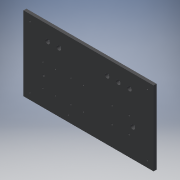
# Autodesk Inventor part: Base2
Saved by Autodesk Inventor 2016 SP1 (Build 200210100, 210)
## iProperties
Created: 2015-09-24
Part Number: Base2
Material: PVC, non plastifié
Document SubType Name: Modeling
Designer: sd
Density: 1.4 g/cm^3
Appearance: Gris
Mass: 783.12 g
Surface Area: 1491.46 cm^2
Volume: 559.372 cm^3
Author: sd
Autodesk Inventor part; units mm, degrees
ref_plane "YZ Plane" through (0, 0, 0) normal (1, 0, 0) x (0, 1, 0)
ref_plane "XZ Plane" through (0, 0, 0) normal (0, 1, 0) x (-1, 0, 0)
ref_plane "XY Plane" through (0, 0, 0) normal (0, 0, 1) x (1, 0, 0)
sketch "Esquisse1" plane through (0, 0, 0) normal (0, 1, 0) x (-1, 0, 0)
  line L0 (-175, 100) -> (175, 100)
  line L1 (175, 100) -> (175, -100)
  line L2 (175, -100) -> (-175, -100)
  line L3 (-175, -100) -> (-175, 100)
  point P0 (0, 0)
  dimension "d0" = 350
  dimension "d1" = 200
  dimension "d93" = 175
  dimension "d94" = 100
  constraints: 8 end point, 2 parallel, 1 horizontal, 1 perpendicular
  measures "d0" distance of L0.start L0.end
  measures "d1" distance of L2.end L0.start
  measures "d93" horizontal distance of point (0, 0) L1.end
  measures "d94" distance from line of point (0, 0) L2
extrude "Extrusion1" add sketch "Esquisse1" along normal blind 8
sketch "Esquisse2" plane through (0, 8, 0) normal (0, 1, 0) x (1, 0, 0)
  line L0 (175, -100) -> (175, 100) projected
  circle A0 centre (109, 46.5) radius 2.25
  circle A1 centre (63, 46.5) radius 2.25
  circle A2 centre (109, 2.5) radius 2.25
  circle A3 centre (63, 2.5) radius 2.25
  line L1 (-175, -100) -> (175, -100) projected
  point P0 (0, 0)
  dimension "d4" = 4.5
  dimension "d5" = 4.5
  dimension "d6" = 4.5
  dimension "d7" = 4.5
  dimension "d14" = 66
  dimension "d15" = 66
  dimension "d46" = 112
  dimension "d47" = 112
  dimension "d48" = 146.5
  dimension "d49" = 146.5
  dimension "d50" = 102.5
  dimension "d51" = 102.5
  constraints: 4 centre point
  measures "d4" diameter of A1
  measures "d5" diameter of A0
  measures "d6" diameter of A2
  measures "d7" diameter of A3
  measures "d14" distance from line of L0 A0.centre
  measures "d15" distance from line of L0 A2.centre
  measures "d46" distance from line of L0 A3.centre
  measures "d47" distance from line of L0 A1.centre
  measures "d48" distance from line of L1 A0.centre
  measures "d49" distance from line of L1 A1.centre
  measures "d50" distance from line of L1 A2.centre
  measures "d51" distance from line of L1 A3.centre
extrude "Extrusion2" cut sketch "Esquisse2" against normal through all
sketch "Esquisse3" plane through (0, 8, 0) normal (0, 1, 0) x (1, 0, 0)
  circle A0 centre (63, 46.5) radius 2.25 projected
  circle A1 centre (63, 2.5) radius 2.25 projected
  line L0 (175, 100) -> (-175, 100) projected
  circle A2 centre (-14, 55.5) radius 2
  circle A3 centre (-48, 55.5) radius 2
  circle A4 centre (-89.1, 55.5) radius 2
  circle A5 centre (-123.1, 55.5) radius 2
  circle A6 centre (-123.1, -6.5) radius 2
  circle A7 centre (-89.1, -6.5) radius 2
  circle A8 centre (-48, -6.5) radius 2
  circle A9 centre (-14, -6.5) radius 2
  point P0 (0, 0)
  dimension "d18" = 4
  dimension "d19" = 4
  dimension "d20" = 4
  dimension "d21" = 4
  dimension "d22" = 4
  dimension "d23" = 4
  dimension "d24" = 4
  dimension "d25" = 4
  dimension "d26" = 62
  dimension "d27" = 62
  dimension "d28" = 62
  dimension "d29" = 62
  dimension "d30" = 34
  dimension "d31" = 34
  dimension "d32" = 34
  dimension "d33" = 34
  dimension "d34" = 41.1
  dimension "d35" = 41.1
  dimension "d36" = 77
  dimension "d37" = 77
  dimension "d38" = 53.5
  dimension "d39" = 44
  dimension "d40" = 44.5
  dimension "d41" = 44.5
  dimension "d42" = 44.5
  dimension "d43" = 44.5
  constraints: 8 centre point
  measures "d18" diameter of A5
  measures "d19" diameter of A4
  measures "d20" diameter of A3
  measures "d21" diameter of A2
  measures "d22" diameter of A9
  measures "d23" diameter of A8
  measures "d24" diameter of A7
  measures "d25" diameter of A6
  measures "d26" distance of A9.centre A2.centre
  measures "d27" distance of A8.centre A3.centre
  measures "d28" distance of A7.centre A4.centre
  measures "d29" distance of A6.centre A5.centre
  measures "d30" distance of A2.centre A3.centre
  measures "d31" distance of A9.centre A8.centre
  measures "d32" distance of A5.centre A4.centre
  measures "d33" distance of A7.centre A6.centre
  measures "d34" distance of A3.centre A4.centre
  measures "d35" distance of A8.centre A7.centre
  measures "d36" horizontal distance of A0.centre A2.centre
  measures "d37" horizontal distance of A1.centre A9.centre
  measures "d38" distance from line of L0 A0.centre
  measures "d39" distance of A1.centre A0.centre
  measures "d40" distance from line of A2.centre L0
  measures "d41" distance from line of L0 A3.centre
  measures "d42" distance from line of L0 A4.centre
  measures "d43" distance from line of L0 A5.centre
extrude "Extrusion3" cut sketch "Esquisse3" against normal through all contours A2 | A3 | A4 | A5 | A6 | A7 | A8 | A9
sketch "Esquisse4" plane through (0, 8, 0) normal (0, 1, 0) x (1, 0, 0)
  circle A0 centre (-121.1, 24.5) radius 3
  circle A1 centre (119, 24.5) radius 6
  circle A2 centre (158, -83) radius 2
  circle A3 centre (158, 83) radius 2
  circle A4 centre (-158, 83) radius 2
  circle A5 centre (-158, -83) radius 2.2714
  circle A6 centre (-110, -60) radius 6
  circle A7 centre (-80, -60) radius 6
  circle A8 centre (50, -60) radius 6
  circle A9 centre (80, -60) radius 6
  circle A10 centre (110, -60) radius 6
  circle A11 centre (-55, 83) radius 2
  line L0 (175, -100) -> (175, 100) projected
  line L1 (-175, 100) -> (-175, -100) projected
  line L2 (175, 100) -> (-175, 100) projected
  line L3 (-175, -100) -> (175, -100) projected
  circle A12 centre (-123.1, 55.5) radius 2 projected
  circle A13 centre (-123.1, -6.5) radius 2 projected
  circle A14 centre (109, 2.5) radius 2.25 projected
  circle A15 centre (109, 46.5) radius 2.25 projected
  point P0 (0, 0)
  dimension "d52" = 4
  dimension "d53" = 4.5428
  dimension "d54" = 4
  dimension "d56" = 4
  dimension "d57" = 6
  dimension "d58" = 12
  dimension "d59" = 17
  dimension "d60" = 17
  dimension "d61" = 17
  dimension "d62" = 17
  dimension "d63" = 17
  dimension "d64" = 17
  dimension "d65" = 17
  dimension "d66" = 4
  dimension "d67" = 17
  dimension "d68" = 2
  dimension "d69" = 31
  dimension "d70" = 62
  dimension "d71" = 17
  dimension "d72" = 120
  dimension "d73" = 44
  dimension "d74" = 22
  dimension "d75" = 10
  dimension "d76" = 30
  dimension "d77" = 12
  dimension "d78" = 12
  dimension "d79" = 12
  dimension "d80" = 12
  dimension "d81" = 12
  dimension "d82" = 30
  dimension "d83" = 30
  dimension "d84" = 40
  dimension "d85" = 40
  dimension "d86" = 40
  dimension "d87" = 65
  dimension "d88" = 40
  dimension "d89" = 40
  dimension "d90" = 130
  constraints: 12 centre point
  measures "d52" diameter of A4
  measures "d53" diameter of A5
  measures "d54" diameter of A3
  measures "d56" diameter of A11
  measures "d57" diameter of A0
  measures "d58" diameter of A1
  measures "d59" distance from line of L1 A4.centre
  measures "d60" distance from line of L2 A4.centre
  measures "d61" distance from line of L2 A3.centre
  measures "d62" distance from line of L0 A3.centre
  measures "d63" distance from line of L1 A5.centre
  measures "d64" distance from line of L3 A5.centre
  measures "d65" distance from line of L3 A2.centre
  measures "d66" diameter of A2
  measures "d67" distance from line of L0 A2.centre
  measures "d68" horizontal distance of A12.centre A0.centre
  measures "d69" vertical distance of A12.centre A0.centre
  measures "d70" distance of A13.centre A12.centre
  measures "d71" distance from line of L2 A11.centre
  measures "d72" distance from line of L1 A11.centre
  measures "d73" distance of A14.centre A15.centre
  measures "d74" vertical distance of A1.centre A15.centre
  measures "d75" horizontal distance of A1.centre A15.centre
  measures "d76" distance of A7.centre A6.centre
  measures "d77" diameter of A6
  measures "d78" diameter of A7
  measures "d79" diameter of A8
  measures "d80" diameter of A9
  measures "d81" diameter of A10
  measures "d82" distance of A9.centre A8.centre
  measures "d83" distance of A10.centre A9.centre
  measures "d84" distance from line of L3 A6.centre
  measures "d85" distance from line of L3 A8.centre
  measures "d86" distance from line of L3 A10.centre
  measures "d87" distance from line of L1 A6.centre
  measures "d88" distance from line of L3 A7.centre
  measures "d89" distance from line of L3 A9.centre
  measures "d90" distance of A7.centre A8.centre
extrude "Extrusion4" cut sketch "Esquisse4" against normal blind 10 contours A0 | A1 | A2 | A3 | A4 | A5 | A6 | A7 | A8 | A9 | A10 | A11
equation "\"d93\" = 0.5 * d0"
equation "\"d94\" = 0.5 * d1"
equation "\"d5\" = d4"
equation "\"d6\" = d4"
equation "\"d7\" = d4"
equation "\"d15\" = d14"
equation "\"d46\" = d47"
equation "\"d49\" = d48"
equation "\"d51\" = d50"
equation "\"d19\" = d18"
equation "\"d20\" = d18"
equation "\"d21\" = d18"
equation "\"d22\" = d18"
equation "\"d23\" = d18"
equation "\"d24\" = d18"
equation "\"d25\" = d18"
equation "\"d27\" = d26"
equation "\"d28\" = d26"
equation "\"d29\" = d26"
equation "\"d31\" = d30"
equation "\"d33\" = d32"
equation "\"d35\" = d34"
equation "\"d37\" = d36"
equation "\"d40\" = d38 + 0.5 * d39 - 0.5 * d26"
equation "\"d41\" = d40"
equation "\"d42\" = d40"
equation "\"d43\" = d40"
equation "\"d54\" = d52"
equation "\"d56\" = d52"
equation "\"d60\" = d59"
equation "\"d61\" = d59"
equation "\"d62\" = d59"
equation "\"d63\" = d59"
equation "\"d64\" = d59"
equation "\"d65\" = d59"
equation "\"d66\" = d52"
equation "\"d67\" = d59"
equation "\"d69\" = 0.5 * d70"
equation "\"d71\" = d59"
equation "\"d74\" = 0.5 * d73"
equation "\"d78\" = d77"
equation "\"d79\" = d77"
equation "\"d80\" = d77"
equation "\"d81\" = d77"
equation "\"d82\" = d76"
equation "\"d83\" = d76"
equation "\"d85\" = d84"
equation "\"d86\" = d85"
equation "\"d88\" = d84"
equation "\"d89\" = d85"
